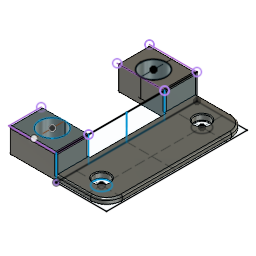
MacBook Pro Front Ear (Autodesk Fusion 360 design; units mm, degrees)
part number: 2025-11-01-16-26-23-759
Autodesk Fusion 360 part; units mm, degrees
sketch "Sketch1" plane through (0, 0, 0) normal (0, 0, 1) x (1, 0, 0)
  line L0 (0, 0) -> (15.875, 0)
  line L1 (15.875, 0) -> (15.875, 44.45)
  line L2 (15.875, 44.45) -> (0, 44.45)
  line L3 (0, 44.45) -> (0, 0)
  circle A0 centre (7.9375, 6.35) radius 2.4
  line L4 (7.9375, 44.45) -> (7.9375, 0) construction
  line L5 (0, 6.35) -> (15.875, 6.35) construction
  line L6 (0, 22.225) -> (15.875, 22.225) construction
  circle A1 centre (7.9375, 6.35) radius 2.4
  line L7 (15.875, 38.1) -> (0, 38.1) construction
  circle A2 centre (7.9375, 38.1) radius 2.4
  dimension "d1" = 15.875
  dimension "d2" = 44.45
  dimension "d5" = 6.35
  dimension "d6" = 15.875
  dimension "d7" = 4.8
  dimension "d9" = 15.875
  dimension "d10" = 4.8
  constraint horizontal L0
  constraint vertical L1
  constraint horizontal L2
  constraint vertical L3
  constraint coincident L0.start L3.end
  constraint midpoint L2 L4.start
  constraint midpoint L0 L4.end
  constraint coincident A0.centre L4
  constraint coincident L3 L5.start
  constraint coincident L1 L5.end
  constraint perpendicular L1 L5
  constraint midpoint A0.centre L5
  constraint coincident L3 L6.start
  constraint coincident L1 L6.end
  constraint perpendicular L1 L6
  constraint coincident L1 L7.start
  constraint coincident L3 L7.end
  constraint midpoint L7 A2.centre
  measures "d1" distance of L0.start L0.end
  measures "d2" distance of L0.start L2.end
  measures "d5" distance of L0 L5
  measures "d6" distance of L5 L6
  measures "d7" diameter of A1
  measures "d9" distance of L6 L7
  measures "d10" diameter of A2
extrude "Extrude1" add sketch "Sketch1" along normal blind 2
sketch "Sketch2" plane through (0, 0, 0) normal (-1, 0, 0) x (0, -1, 0)
  line L0 (-44.45, 0) -> (0, 0)
  line L1 (0, 0) -> (0, 2)
  line L2 (0, 2) -> (-44.45, 2)
  line L3 (-44.45, 2) -> (-44.45, 0)
  line L4 (-44.45, 0) -> (0, 0)
  line L5 (0, 0) -> (0, 8)
  line L6 (0, 8) -> (-44.45, 8)
  line L7 (-44.45, 8) -> (-44.45, 0)
  line L8 (-22.225, 0) -> (-22.225, 8) construction
  line L9 (-22.225, 8) -> (-10.225, 8)
  line L10 (-10.225, 8) -> (-10.225, 0)
  line L11 (-10.225, 0) -> (-22.225, 0)
  line L12 (-22.225, 0) -> (-22.225, 8)
  line L13 (-22.225, 8) -> (-34.225, 8)
  line L14 (-34.225, 8) -> (-34.225, 0)
  line L15 (-34.225, 0) -> (-22.225, 0)
  line L16 (-22.225, 0) -> (-22.225, 8)
  dimension "d13" = 8
  dimension "d14" = 12
  dimension "d15" = 12
  constraint horizontal L4
  constraint vertical L5
  constraint horizontal L6
  constraint vertical L7
  constraint coincident L0.start L3.end
  constraint midpoint L0 L8.start
  constraint midpoint L6 L8.end
  constraint horizontal L9
  constraint vertical L10
  constraint horizontal L11
  constraint vertical L12
  constraint horizontal L13
  constraint vertical L14
  constraint horizontal L15
  constraint vertical L16
  measures "d13" distance of L0.start L6.end
  measures "d14" distance of L8.end L9.end
  measures "d15" distance of L8.end L13.end
extrude "Extrude2" add sketch "Sketch2" along normal blind 15 contours L0 L2 L3 L4 L7 L14 | L2 L6 L7 L14 | L0 L1 L2 L4 L5 L10 | L2 L5 L6 L10
fillet "Outer Edge Fillet" radius 5 2 edges at (15.875, 0, 1) (15.875, 44.45, 1)
sketch "Sketch4" plane through (0, 0, 8) normal (0, 0, 1) x (-1, 0, 0)
  line L0 (0, -10.225) -> (15, -10.225)
  line L1 (7.5, -10.225) -> (7.5, -0.5) construction
  circle A0 centre (7.5, -6.225) radius 4
  line L2 (15, -10.225) -> (15, 0)
  line L3 (0, 0) -> (0, -10.225)
  line L4 (15, 0) -> (0, 0)
  line L5 (0, -34.225) -> (15, -34.225)
  line L6 (0, -44.45) -> (15, -44.45)
  line L7 (7.5, -34.225) -> (7.5, -44.45) construction
  circle A1 centre (7.5, -38.225) radius 4
  dimension "d37" = 8
  dimension "d41" = 8
  constraint midpoint L0 L1.start
  constraint coincident L1 A0.centre
  constraint tangent L0 A0
  constraint midpoint L5 L7.start
  constraint midpoint L6 L7.end
  constraint coincident L7 A1.centre
  constraint tangent L5 A1
  measures "d37" diameter of A0
  measures "d41" diameter of A1
extrude "Extrude5" cut sketch "Sketch4" against normal blind 6 contours A0 | A1
fillet "Fillet2" radius 0.5 30 edges at (5.4375, 0, 2) (14.4105, 1.4645, 2) (15.875, 22.225, 2) (14.4105, 42.9855, 2) (5.4375, 44.45, 2) (-2.0625, 0, 0) (14.4105, 1.4645, 0) (15.875, 22.225, 0) (14.4105, 42.9855, 0) (-2.0625, 44.45, 0) (-15, 5.1125, 0) (0, 22.225, 0) (0, 22.225, 2) (-7.5, 34.225, 0) (-15, 34.225, 4) (-15, 39.3375, 0) (-15, 39.3375, 8) (0, 39.3375, 8) (0, 34.225, 5) (-7.5, 44.45, 8) (-15, 44.45, 4) (0, 44.45, 5) (-15, 0, 4) (0, 0, 5) (-7.5, 0, 8) (0, 5.1125, 8) (-15, 5.1125, 8) (-15, 10.225, 4) (0, 10.225, 5) (-7.5, 10.225, 0)
fillet "Fillet2" radius 0.25 4 edges at (5.6999, 7.2179, 0) (5.6999, 7.2179, 2) (5.6999, 38.9679, 0) (5.6999, 38.9679, 2)
equation "d1 = bracket_width"
equation "d2 = ru"
equation "d5 = ru_gap"
equation "d6 = hole_spacing"
equation "d7 = hole_diameter"
equation "d9 = hole_spacing"
equation "d10 = hole_diameter"
equation "d11 = thickness"
equation "d13 = front_depth + thickness"
equation "d14 = laptop_thickness / 2"
equation "d15 = laptop_thickness / 2"
equation "d16 = ear_width"
equation "thickness = 2 mm"
equation "laptop_thickness = 24 mm"
equation "hole_diameter = 4.8 mm"
equation "ru_gap = 6.35 mm"
equation "hole_spacing = 15.875 mm"
equation "ru = 44.45 mm"
equation "bracket_width = 15.875 mm"
equation "ear_width = 15 mm"
equation "rod_diameter = 8 mm"
equation "extension_length = 90 mm"
equation "d37 = rod_diameter"
equation "front_depth = 6 mm"
equation "d41 = rod_diameter"
equation "d44 = -front_depth"
named bodies: "Front Ear"
